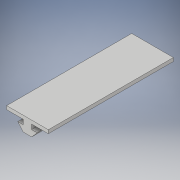
# Autodesk Inventor part: railMount_4.5inch
Saved by Autodesk Inventor 2018 (Build 220112000, 112)
## iProperties
Created: 2020-03-10
Part Number: railMount_4.5inch
Material: Generic
Document SubType Name: Modeling
Designer: natha
Density: 1 g/cm^3
Appearance: Default
Author: natha
Autodesk Inventor part; units mm, degrees
ref_plane "YZ Plane" through (0, 0, 0) normal (1, 0, 0) x (0, 1, 0)
ref_plane "XZ Plane" through (0, 0, 0) normal (0, 1, 0) x (-1, 0, 0)
ref_plane "XY Plane" through (0, 0, 0) normal (0, 0, 1) x (1, 0, 0)
sketch "Sketch1" plane through (0, 0, 0) normal (0, 1, 0) x (-1, 0, 0)
  line L0 (0, 0) -> (38.1, 0)
  line L1 (38.1, 0) -> (38.1, -114.3)
  line L2 (38.1, -114.3) -> (0, -114.3)
  line L3 (0, -114.3) -> (0, 0)
  dimension "d0" = 38.1
  dimension "d1" = 114.3
  constraints: 8 end point, 2 parallel, 1 horizontal, 1 perpendicular
  measures "d0" distance of L1.end L2.end
  measures "d1" distance of L0.end L1.end
extrude "Extrusion1" add sketch "Sketch1" along normal blind 3.175
sketch "Sketch2" plane through (-38.1, 0, 0) normal (0, 0, 1) x (1, 0, 0)
  line L0 (38.1, 0) -> (0, 0) projected
  line L1 (15.24, 0) -> (15.24, -4.318)
  line L2 (22.86, -4.318) -> (22.86, 0)
  line L3 (15.24, 0) -> (22.86, 0)
  line L4 (0, 0) -> (0, 3.175) projected
  line L5 (38.1, 0) -> (38.1, 3.175) projected
  line L6 (22.86, -4.318) -> (27.94, -4.318)
  line L7 (15.24, -4.318) -> (10.16, -4.318)
  line L8 (10.16, -4.318) -> (15.24, -10.16)
  line L9 (15.24, -10.16) -> (22.86, -10.16)
  line L10 (22.86, -10.16) -> (27.94, -4.318)
  dimension "d4" = 15.24
  dimension "d5" = 15.24
  dimension "d7" = 5.08
  dimension "d8" = 5.08
  dimension "d9" = 7.62
  dimension "d10" = 10.16
  constraints: 16 end point, 2 horizontal, 2 point on line, 1 parallel, 1 perpendicular, 1 vertical
  measures "d4" distance between parallel lines of L4 L1
  measures "d5" distance between parallel lines of L5 L2
  measures "d7" distance of L2.start L6.end
  measures "d8" distance of L1.end L7.end
  measures "d9" distance of L8.end L9.end
  measures "d10" distance between parallel lines of L0 L9
extrude "Extrusion2" add sketch "Sketch2" against normal blind 114.3
body "Solid1"
